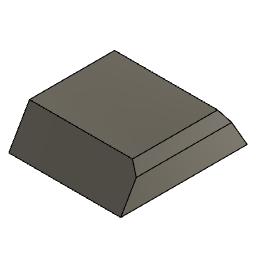
Dovetail Cap v1 (Autodesk Fusion 360 design; units mm, degrees)
Autodesk Fusion 360 part; units mm, degrees
sketch "Sketch1" plane through (0, 0, 0) normal (1, 0, 0) x (0, 1, 0)
  line L0 (0, 0) -> (2.3094, 4)
  line L1 (2.3094, 4) -> (11.8094, 4)
  line L2 (11.8094, 4) -> (14.1188, 0)
  line L3 (14.1188, 0) -> (0, 0)
  dimension "d1" = 4
  dimension "d2" = 9.5
  dimension "d3" = 60
  constraint coincident L0.start L3.end
  constraint horizontal L1
  constraint parallel L1 L3
  constraint equal L0 L2
  measures "d1" vertical distance of L0.start L0.end
  measures "d2" distance of L0.end L1.end
  measures "d3" angle of L0 L3
extrude "Extrude1" add sketch "Sketch1" along normal blind 12.5
chamfer "Chamfer1" distance 1 angle 45 1 edges at (12.5, 7.0594, 4)
